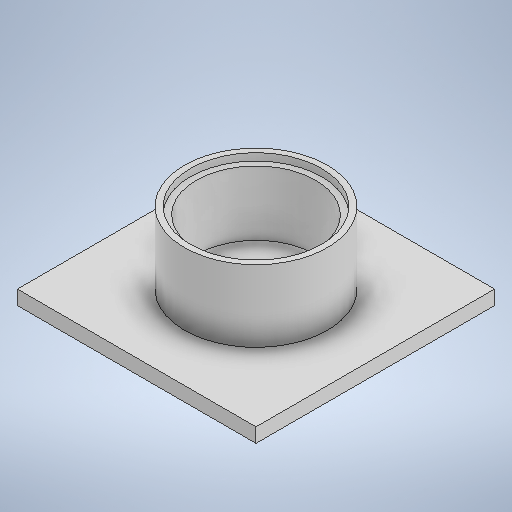
# Autodesk Inventor part: 1
Saved by Autodesk Inventor 2025.1 (Build 291241020, 241B)
## iProperties
Created: 2024-11-01
Part Number: 1
Material: Generic
Document SubType Name: Modeling
Designer: Krishnu
Density: 1 g/cm^3
Appearance: Default
Author: Krishnu
Autodesk Inventor part; units mm, degrees
ref_plane "YZ Plane" through (0, 0, 0) normal (1, 0, 0) x (0, 1, 0)
ref_plane "XZ Plane" through (0, 0, 0) normal (0, 1, 0) x (-1, 0, 0)
ref_plane "XY Plane" through (0, 0, 0) normal (0, 0, 1) x (1, 0, 0)
sketch "Sketch1" plane through (0, 0, 0) normal (0, 1, 0) x (-1, 0, 0)
  circle A0 centre (0, 0) radius 317.5
  circle A1 centre (0, 0) radius 380.1959
  dimension "d0" = 635
  dimension "d1" = 760.3918
  constraints: 2 centre point, 2 coincident
  measures "d0" diameter of A0
  measures "d1" diameter of A1
extrude "Extrusion1" add sketch "Sketch1" along normal blind 381
sketch "Sketch2" plane through (0, 0, 0) normal (0, -1, 0) x (1, 0, 0)
  line L0 (635, 635) -> (-635, 635)
  line L1 (-635, 635) -> (-635, -635)
  line L2 (-635, -635) -> (635, -635)
  line L3 (635, -635) -> (635, 635)
  circle A0 centre (0, 0) radius 380.1959 projected
  dimension "d4" = 635
  dimension "d5" = 635
  dimension "d6" = 635
  dimension "d7" = 635
  constraints: 8 end point, 2 parallel, 1 horizontal, 1 perpendicular
  measures "d4" distance from line of L2 A0.centre
  measures "d5" distance from line of L3 A0.centre
  measures "d6" distance from line of L0 A0.centre
  measures "d7" distance from line of L1 A0.centre
extrude "Extrusion2" add sketch "Sketch2" along normal blind 76.2 contours L3 L2 L1 L0 | A0
sketch "Sketch3" plane through (0, 381, 0) normal (0, 1, 0) x (1, 0, 0)
  circle A0 centre (0, 0) radius 349.7159
  circle A1 centre (0, 0) radius 380.1959 projected
  circle A2 centre (0, 0) radius 317.5 projected
  dimension "d10" = 30.48
  dimension "d11" = 760.3918
  dimension "d12" = 32.2159
  constraints: 1 centre point, 1 coincident
  measures "d10" radial gap between concentric circles of A1 A0
  measures "d11" diameter of A1
  measures "d12" radial gap between concentric circles of A0 A2
extrude "Extrusion3" cut sketch "Sketch3" against normal blind 38.1 contours A0 | A2
body "Solid1"
